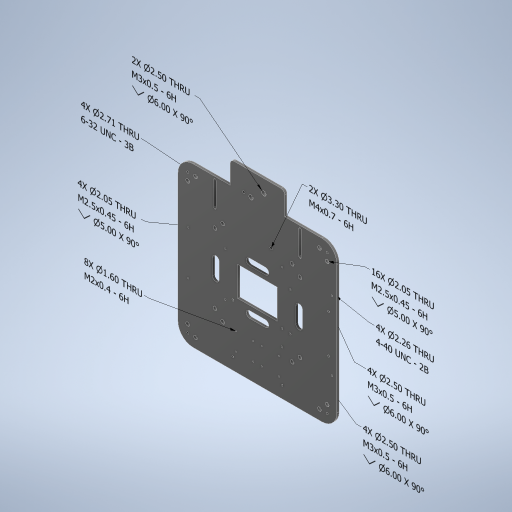
# Autodesk Inventor part: phase_payload_bay_redo_in_inventor_for_danny
Saved by Autodesk Inventor 2023.2 (Build 272271030, 271C)
## iProperties
Created: 2023-02-10
Part Number: phase_payload_bay_redo_in_inventor_for_danny
Material: ABS Plastic
Document SubType Name: Modeling
Designer: makhi
Density: 1.06 g/cm^3
Appearance: Smooth - White
Author: makhi
Autodesk Inventor part; units mm, degrees
ref_plane "YZ Plane" through (0, 0, 0) normal (1, 0, 0) x (0, 1, 0)
ref_plane "XZ Plane" through (0, 0, 0) normal (0, 1, 0) x (-1, 0, 0)
ref_plane "XY Plane" through (0, 0, 0) normal (0, 0, 1) x (1, 0, 0)
sketch "Bay outline: sketch" plane through (0, 0, 0) normal (0, 0, 1) x (1, 0, 0)
  line L0 (105, 84.9999) -> (105, -84.9999)
  line L1 (85, -104.9999) -> (-85, -104.9999)
  line L2 (-105, -84.9999) -> (-105, 84.9999)
  line L3 (-31.0001, 135.0001) -> (31.0001, 135.0001)
  line L4 (36.0001, 130.0001) -> (36.0001, 104.9999)
  line L5 (-36.0001, 104.9999) -> (-36.0001, 130.0001)
  arc A0 (-85, 104.9999) -> (-105, 84.9999) centre (-85, 84.9999) ccw
  arc A1 (105, 84.9999) -> (85, 104.9999) centre (85, 84.9999) ccw
  arc A2 (85, -104.9999) -> (105, -84.9999) centre (85, -84.9999) ccw
  arc A3 (-105, -84.9999) -> (-85, -104.9999) centre (-85, -84.9999) ccw
  arc A4 (-31.0001, 135.0001) -> (-36.0001, 130.0001) centre (-31.0001, 130.0001) ccw
  arc A5 (36.0001, 130.0001) -> (31.0001, 135.0001) centre (31.0001, 130.0001) ccw
  line L6 (-36.0001, 104.9999) -> (-85, 104.9999)
  line L7 (36.0001, 104.9999) -> (85, 104.9999)
  dimension "d0" = 20
  dimension "d1" = 5
  constraints: 16 end point, 12 point on circle, 10 tangent, 6 centre point, 4 equal radius, 3 equal length, 2 horizontal, 1 perpendicular
  measures "d0" radius of A0
  measures "d1" radius of A4
extrude "Extrusion1" add sketch "Bay outline: sketch" along normal blind 3
sketch "Cutouts for balun, cables and splitter" plane through (0, 0, 3) normal (0, 0, 1) x (1, 0, 0)
  line L0 (56.2059, 102.5001) -> (56.2061, 102.5001)
  line L1 (57.7061, 101.0001) -> (57.7061, 68.9999)
  line L2 (56.2061, 67.4999) -> (56.2059, 67.4999)
  line L3 (54.7059, 68.9999) -> (54.7059, 101.0001)
  arc A0 (56.2059, 102.5001) -> (54.7059, 101.0001) centre (56.2059, 101.0001) ccw
  arc A1 (57.7061, 101.0001) -> (56.2061, 102.5001) centre (56.2061, 101.0001) ccw
  arc A2 (56.2061, 67.4999) -> (57.7061, 68.9999) centre (56.2061, 68.9999) ccw
  arc A3 (54.7059, 68.9999) -> (56.2059, 67.4999) centre (56.2059, 68.9999) ccw
  line L4 (-56.2061, 102.5001) -> (-56.2059, 102.5001)
  line L5 (-54.7059, 101.0001) -> (-54.7059, 68.9999)
  line L6 (-56.2059, 67.4999) -> (-56.2061, 67.4999)
  line L7 (-57.7061, 68.9999) -> (-57.7061, 101.0001)
  arc A4 (-56.2061, 102.5001) -> (-57.7061, 101.0001) centre (-56.2061, 101.0001) ccw
  arc A5 (-54.7059, 101.0001) -> (-56.2059, 102.5001) centre (-56.2059, 101.0001) ccw
  arc A6 (-56.2059, 67.4999) -> (-54.7059, 68.9999) centre (-56.2059, 68.9999) ccw
  arc A7 (-57.7061, 68.9999) -> (-56.2061, 67.4999) centre (-56.2061, 68.9999) ccw
  line L8 (-26.2, 19.5001) -> (26.2, 19.5001)
  line L9 (26.2, 19.5001) -> (26.2, -19.5001)
  line L10 (26.2, -19.5001) -> (-26.2, -19.5001)
  line L11 (-26.2, -19.5001) -> (-26.2, 19.5001)
  line L12 (54.9998, 14.9998) -> (55.0002, 14.9998)
  line L13 (59.5002, 10.4998) -> (59.5002, -10.4998)
  line L14 (55.0002, -14.9998) -> (54.9998, -14.9998)
  line L15 (50.4998, -10.4998) -> (50.4998, 10.4998)
  arc A8 (54.9998, 14.9998) -> (50.4998, 10.4998) centre (54.9998, 10.4998) ccw
  arc A9 (59.5002, 10.4998) -> (55.0002, 14.9998) centre (55.0002, 10.4998) ccw
  arc A10 (55.0002, -14.9998) -> (59.5002, -10.4998) centre (55.0002, -10.4998) ccw
  arc A11 (50.4998, -10.4998) -> (54.9998, -14.9998) centre (54.9998, -10.4998) ccw
  line L16 (-55.0002, 14.9998) -> (-54.9998, 14.9998)
  line L17 (-50.4998, 10.4998) -> (-50.4998, -10.4998)
  line L18 (-54.9998, -14.9998) -> (-55.0002, -14.9998)
  line L19 (-59.5002, -10.4998) -> (-59.5002, 10.4998)
  arc A12 (-55.0002, 14.9998) -> (-59.5002, 10.4998) centre (-55.0002, 10.4998) ccw
  arc A13 (-50.4998, 10.4998) -> (-54.9998, 14.9998) centre (-54.9998, 10.4998) ccw
  arc A14 (-54.9998, -14.9998) -> (-50.4998, -10.4998) centre (-54.9998, -10.4998) ccw
  arc A15 (-59.5002, -10.4998) -> (-55.0002, -14.9998) centre (-55.0002, -10.4998) ccw
  line L20 (-14.9998, 29.9998) -> (-14.9998, 30.0002)
  line L21 (-10.4998, 34.5002) -> (10.4998, 34.5002)
  line L22 (14.9998, 30.0002) -> (14.9998, 29.9998)
  line L23 (10.4998, 25.4998) -> (-10.4998, 25.4998)
  arc A16 (-14.9998, 29.9998) -> (-10.4998, 25.4998) centre (-10.4998, 29.9998) ccw
  arc A17 (-10.4998, 34.5002) -> (-14.9998, 30.0002) centre (-10.4998, 30.0002) ccw
  arc A18 (14.9998, 30.0002) -> (10.4998, 34.5002) centre (10.4998, 30.0002) ccw
  arc A19 (10.4998, 25.4998) -> (14.9998, 29.9998) centre (10.4998, 29.9998) ccw
  line L24 (-14.9998, -30.0002) -> (-14.9998, -29.9998)
  line L25 (-10.4998, -25.4998) -> (10.4998, -25.4998)
  line L26 (14.9998, -29.9998) -> (14.9998, -30.0002)
  line L27 (10.4998, -34.5002) -> (-10.4998, -34.5002)
  arc A20 (-14.9998, -30.0002) -> (-10.4998, -34.5002) centre (-10.4998, -30.0002) ccw
  arc A21 (-10.4998, -25.4998) -> (-14.9998, -29.9998) centre (-10.4998, -29.9998) ccw
  arc A22 (14.9998, -29.9998) -> (10.4998, -25.4998) centre (10.4998, -29.9998) ccw
  arc A23 (10.4998, -34.5002) -> (14.9998, -30.0002) centre (10.4998, -30.0002) ccw
  point P0 (55, 0)
  point P1 (-55, 0)
  point P2 (0, 30)
  point P3 (0, -30)
  dimension "d5" = 1.5
  dimension "d6" = 1.5
  dimension "d8" = 4.5
  dimension "d9" = 4.5
  dimension "d10" = 4.5
  dimension "d11" = 4.5
  constraints: 56 end point, 48 point on circle, 48 tangent, 24 centre point, 18 equal radius, 14 parallel, 7 perpendicular, 5 horizontal
  measures "d5" radius of A0
  measures "d6" radius of A4
  measures "d8" radius of A8
  measures "d9" radius of A12
  measures "d10" radius of A16
  measures "d11" radius of A20
sketch "Antenna mount holes" plane through (0, 0, 3) normal (0, 0, 1) x (1, 0, 0)
  circle A0 centre (45.873, 56.127) radius 1.2499
  circle A1 centre (-45.873, 56.127) radius 1.2499
  circle A2 centre (45.873, -56.127) radius 1.2499
  circle A3 centre (-45.873, -56.127) radius 1.2499
  circle A4 centre (56.127, 45.873) radius 1.2499
  circle A5 centre (-56.127, 45.873) radius 1.2499
  circle A6 centre (56.127, -45.873) radius 1.2499
  circle A7 centre (-56.127, -45.873) radius 1.2499
  circle A8 centre (81.873, 92.127) radius 1.2499
  circle A9 centre (-81.873, 92.127) radius 1.2499
  circle A10 centre (81.873, -92.127) radius 1.2499
  circle A11 centre (-81.873, -92.127) radius 1.2499
  circle A12 centre (92.127, 81.873) radius 1.2499
  circle A13 centre (-92.127, 81.873) radius 1.2499
  circle A14 centre (92.127, -81.873) radius 1.2499
  circle A15 centre (-92.127, -81.873) radius 1.2499
  constraints: 16 centre point
sketch "#6 standoff holes" plane through (0, 0, 0) normal (0, 0, 1) x (1, 0, 0)
  circle A0 centre (92, 92) radius 1.8984
  circle A1 centre (-92, 92) radius 1.8984
  circle A2 centre (92, -92) radius 1.8984
  circle A3 centre (-92, -92) radius 1.8984
  constraints: 4 centre point
hole "Hole2" at (92, 92, 0) at (-92, 92, 0) at (-92, -92, 0) at (92, -92, 0) direction (0, 0, 1) diameter 2.6416 end through all thread size "6-32 UNC" class "3B" standard "ANSI Unified Screw Threads"
hole "Hole5" at (45.873, 56.127, 3) at (56.127, 45.873, 3) at (92.127, 81.873, 3) at (81.873, 92.127, 3) at (-92.127, 81.873, 3) at (-81.873, 92.127, 3) at (-45.873, 56.127, 3) at (-56.127, 45.873, 3) at (-45.873, -56.127, 3) at (-56.127, -45.873, 3) at (-92.127, -81.873, 3) at (-81.873, -92.127, 3) at (45.873, -56.127, 3) at (56.127, -45.873, 3) at (92.127, -81.873, 3) at (81.873, -92.127, 3) direction (0, 0, -1) diameter 2.013 end through all countersink diameter 5 countersink angle 90 thread size "M2.5x0.45" class "6H" standard "ISO Metric profile"
sketch "Pi mount holes (bottom)" plane through (0, 0, 0) normal (0, 0, -1) x (-1, 0, 0)
  circle A0 centre (91.5, 29) radius 1.2501
  circle A1 centre (42.5, 29) radius 1.2501
  circle A2 centre (42.5, -29) radius 1.2501
  circle A3 centre (91.5, -29) radius 1.2501
  constraints: 4 centre point
hole "Hole6" at (-91.5, 29, 0) at (-91.5, -29, 0) at (-42.5, -29, 0) at (-42.5, 29, 0) direction (0, 0, 1) diameter 2.013 end through all countersink diameter 5 countersink angle 90 thread size "M2.5x0.45" class "6H" standard "ISO Metric profile"
sketch "Switch mount holes" plane through (0, 0, 3) normal (0, 0, 1) x (1, 0, 0)
  circle A0 centre (18, 60) radius 2.0002
  circle A1 centre (-18, 106) radius 2.0002
  constraints: 2 centre point
hole "Hole7" at (18, 60, 3) at (-18, 106, 3) direction (0, 0, -1) diameter 3.242 end through all thread size "M4x0.7" class "6H" standard "ISO Metric profile"
sketch "SONAR mount holes" plane through (0, 0, 3) normal (0, 0, 1) x (1, 0, 0)
  circle A0 centre (-8.501, 105) radius 1.4999
  circle A1 centre (8.519, 117.95) radius 1.4999
  constraints: 2 centre point
hole "Hole8" at (-8.501, 105, 3) at (8.519, 117.95, 3) direction (0, 0, -1) diameter 2.459 end through all countersink diameter 6 countersink angle 90 thread size "M3x0.5" class "6H" standard "ISO Metric profile"
sketch "RFoF mount holes" plane through (0, 0, 0) normal (0, 0, 1) x (1, 0, 0)
  circle A0 centre (32.5, -24.5) radius 1.5
  circle A1 centre (-32.5, -24.5) radius 1.5
  circle A2 centre (32.5, -89.5) radius 1.5
  circle A3 centre (-32.5, -89.5) radius 1.5
  constraints: 4 centre point
hole "Hole9" at (32.5, -24.5, 0) at (-32.5, -24.5, 0) at (-32.5, -89.5, 0) at (32.5, -89.5, 0) direction (0, 0, 1) diameter 2.459 end through all countersink diameter 6 countersink angle 90 thread size "M3x0.5" class "6H" standard "ISO Metric profile"
sketch "Orolia mount holes" plane through (0, 0, 0) normal (0, 0, 1) x (1, 0, 0)
  circle A0 centre (93.98, 25.4) radius 1.5001
  circle A1 centre (43.18, 25.4) radius 1.5001
  circle A2 centre (93.98, -25.4) radius 1.5001
  circle A3 centre (43.18, -25.4) radius 1.5001
  constraints: 4 centre point
hole "Hole10" at (93.98, 25.4, 0) at (43.18, 25.4, 0) at (93.98, -25.4, 0) at (43.18, -25.4, 0) direction (0, 0, 1) diameter 2.459 end through all countersink diameter 6 countersink angle 90 thread size "M3x0.5" class "6H" standard "ISO Metric profile"
sketch "OLED mount holes" plane through (0, 0, 3) normal (0, 0, 1) x (1, 0, 0)
  circle A0 centre (28.4, -58.04) radius 1.0001
  circle A1 centre (5.6, -58.04) radius 1.0001
  circle A2 centre (5.6, -81.54) radius 1.0001
  circle A3 centre (28.4, -81.54) radius 1.0001
  circle A4 centre (-5.6, -58.04) radius 1.0001
  circle A5 centre (-28.4, -58.04) radius 1.0001
  circle A6 centre (-28.4, -81.54) radius 1.0001
  circle A7 centre (-5.6, -81.54) radius 1.0001
  constraints: 8 centre point
hole "Hole11" at (-28.4, -58.04, 3) at (-28.4, -81.54, 3) at (-5.6, -81.54, 3) at (-5.6, -58.04, 3) at (5.6, -81.54, 3) at (5.6, -58.04, 3) at (28.4, -58.04, 3) at (28.4, -81.54, 3) direction (0, 0, -1) diameter 1.567 end through all thread size "M2x0.4" class "6H" standard "ISO Metric profile"
sketch "PRS10 mount holes" plane through (0, 0, 0) normal (0, 0, 1) x (1, 0, 0)
  circle A0 centre (98.552, 45.72) radius 1.4284
  circle A1 centre (32.512, 45.72) radius 1.4284
  circle A2 centre (98.552, -45.72) radius 1.4284
  circle A3 centre (32.512, -45.72) radius 1.4284
  constraints: 4 centre point
hole "Hole12" at (98.552, 45.72, 0) at (32.512, 45.72, 0) at (32.512, -45.72, 0) at (98.552, -45.72, 0) direction (0, 0, 1) diameter 2.1565 end through all thread size "4-40 UNC" class "2B" standard "ANSI Unified Screw Threads"
extrude "Extrusion4" cut sketch "Cutouts for balun, cables and splitter" against normal blind 10
